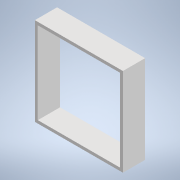
# Autodesk Inventor part: Верх
Saved by Autodesk Inventor 2021.2 (Build 252289000, 289)
## iProperties
Created: 2021-11-01
Part Number: Верх
Material: Типовые
Document SubType Name: Modeling
Designer: Kolan
Density: 1 g/cm^3
Appearance: По умолчанию
Author: Kolan
Autodesk Inventor part; units mm, degrees
ref_plane "YZ Plane" through (0, 0, 0) normal (1, 0, 0) x (0, 1, 0)
ref_plane "XZ Plane" through (0, 0, 0) normal (0, 1, 0) x (-1, 0, 0)
ref_plane "XY Plane" through (0, 0, 0) normal (0, 0, 1) x (1, 0, 0)
sketch "Эскиз1" plane through (0, 0, 0) normal (0, 0, 1) x (1, 0, 0)
  line L0 (41.178, 40.928) -> (-41.178, 40.928) construction
  line L1 (-41.178, 40.928) -> (-41.178, -40.928) construction
  line L2 (-41.178, -40.928) -> (41.178, -40.928) construction
  line L3 (41.178, -40.928) -> (41.178, 40.928) construction
  circle A0 centre (22.7283, 19.0964) radius 1 construction
  circle A1 centre (-19.4499, -22.8747) radius 1 construction
  circle A2 centre (19.3464, -22.9783) radius 1 construction
  line L4 (17.2251, 27.428) -> (22.7282, 21.9249) construction
  line L5 (22.7282, 21.9249) -> (19.8998, 19.0964) construction
  line L6 (19.8998, 19.0964) -> (22.7282, 16.268) construction
  line L7 (22.7282, 16.268) -> (25.5567, 19.0964) construction
  line L8 (25.5567, 19.0964) -> (27.678, 16.9751) construction
  line L9 (27.678, 16.9751) -> (27.678, -17.4751) construction
  line L10 (27.678, -17.4751) -> (22.1749, -22.9783) construction
  line L11 (22.1749, -22.9783) -> (19.3464, -20.1498) construction
  line L12 (19.3464, -20.1498) -> (16.518, -22.9783) construction
  line L13 (16.518, -22.9783) -> (19.3464, -25.8067) construction
  line L14 (19.3464, -25.8067) -> (17.2251, -27.928) construction
  line L15 (17.2251, -27.928) -> (-17.2251, -27.928) construction
  line L16 (-17.2251, -27.928) -> (-19.3464, -25.8067) construction
  line L17 (-19.3464, -25.8067) -> (-16.518, -22.9783) construction
  line L18 (-16.518, -22.9783) -> (-19.3464, -20.1498) construction
  line L19 (-19.3464, -20.1498) -> (-22.1749, -22.9783) construction
  line L20 (-22.1749, -22.9783) -> (-27.678, -17.4751) construction
  line L21 (-27.678, -17.4751) -> (-27.678, 16.9751) construction
  line L22 (-27.678, 16.9751) -> (-17.2251, 27.428) construction
  line L23 (-17.2251, 27.428) -> (17.2251, 27.428) construction
  line L24 (27.678, 27.428) -> (-27.678, 27.428)
  line L25 (-27.678, 27.428) -> (-27.678, -27.928)
  line L26 (-27.678, -27.928) -> (27.678, -27.928)
  line L27 (27.678, -27.928) -> (27.678, 27.428)
  line L28 (29.678, -29.928) -> (-29.678, -29.928)
  line L29 (-29.678, -29.928) -> (-29.678, 29.428)
  line L30 (-29.678, 29.428) -> (29.678, 29.428)
  line L31 (29.678, 29.428) -> (29.678, -29.928)
  point P0 (0, 0)
  dimension "d0" = 2
  constraints: 16 end point, 4 parallel, 2 perpendicular, 1 horizontal, 1 point on line, 3 other
  measures "d0" distance between parallel lines of L26 L28
extrude "Выдавливание1" add sketch "Эскиз1" along normal blind 10
sketch "Эскиз2" plane through (0, 0, 10) normal (0, 0, 1) x (1, 0, 0)
  line L0 (29.678, 29.428) -> (-29.678, 29.428) projected
  line L1 (-29.678, 29.428) -> (-29.678, -29.928) projected
  line L2 (29.678, 29.428) -> (-29.678, 29.428)
  line L3 (-29.678, 29.428) -> (-29.678, -29.928)
  line L4 (-29.678, -29.928) -> (29.678, -29.928)
  line L5 (29.678, -29.928) -> (29.678, 29.428)
  point P0 (0, 0)
  constraints: 8 end point, 2 parallel, 1 horizontal, 1 perpendicular
extrude "Выдавливание2" add sketch "Эскиз2" along normal blind 1.5
sketch "Эскиз3" plane through (0, 0, 10) normal (0, 0, -1) x (-1, 0, 0)
  line L0 (-27.678, 27.428) -> (-27.678, -27.928) construction
  line L1 (-27.678, -27.928) -> (27.678, -27.928) construction
  line L2 (27.678, -27.928) -> (27.678, 27.428) construction
  line L3 (27.678, 27.428) -> (-27.678, 27.428) construction
  line L4 (-29.678, -29.928) -> (-29.678, 29.428) construction
  line L5 (-29.678, -3.25) -> (-25.678, -3.25)
  line L6 (-25.678, -3.25) -> (-25.678, 2.75)
  line L7 (-25.678, 2.75) -> (-29.678, 2.75)
  line L8 (-29.678, 2.75) -> (-29.678, -3.25)
  line L9 (-27.678, 27.428) -> (-27.678, -27.928) construction
  line L10 (-27.678, -0.25) -> (27.678, -0.25) construction
  line L11 (0, -27.928) -> (0, 27.428) construction
  line L12 (29.678, -3.25) -> (25.678, -3.25)
  line L13 (25.678, -3.25) -> (25.678, 2.75)
  line L14 (25.678, 2.75) -> (29.678, 2.75)
  line L15 (29.678, 2.75) -> (29.678, -3.25)
  line L16 (-29.678, 29.428) -> (29.678, 29.428) construction
  line L17 (-3, 29.428) -> (3, 29.428)
  line L18 (3, 29.428) -> (3, 25.428)
  line L19 (3, 25.428) -> (-3, 25.428)
  line L20 (-3, 25.428) -> (-3, 29.428)
  line L21 (-3, -29.928) -> (3, -29.928)
  line L22 (3, -29.928) -> (3, -25.928)
  line L23 (3, -25.928) -> (-3, -25.928)
  line L24 (-3, -25.928) -> (-3, -29.928)
  point P0 (0, 0)
  dimension "d5" = 4
  dimension "d6" = 6
  dimension "d7" = 3
  dimension "d8" = 6
  dimension "d9" = 4
  dimension "d10" = 3
  constraints: 36 end point, 8 symmetric about line, 4 midpoint, 4 parallel, 2 horizontal, 2 perpendicular, 2 point on line
  measures "d5" distance of L7.end L6.end
  measures "d6" distance of L6.end L5.end
  measures "d7" distance from line of L10.start L7
  measures "d8" distance of L18.end L19.end
  measures "d9" distance of L17.end L18.end
  measures "d10" distance between parallel lines of L11 L18
extrude "Выдавливание3" add sketch "Эскиз3" along normal blind 20
sketch "Эскиз4" plane through (0, 0, 11.5) normal (0, 0, 1) x (1, 0, 0)
  line L0 (-10, -16.25) -> (5, -16.25)
  line L1 (5, -16.25) -> (5, 15.75)
  line L2 (5, 15.75) -> (-10, 15.75)
  line L3 (-10, 15.75) -> (-10, -16.25)
  line L4 (-29.678, 29.428) -> (-29.678, -29.928) construction
  point P0 (0, 0)
  point P1 (-29.678, -0.25)
  dimension "d13" = 15
  dimension "d14" = 32
  dimension "d15" = 16
  dimension "d16" = 5
  constraints: 8 end point, 2 parallel, 1 horizontal, 1 midpoint, 1 perpendicular
  measures "d13" distance of L2.end L1.end
  measures "d14" distance of L1.end L0.end
  measures "d15" distance from line of point (-29.678, -0.25) L2
  measures "d16" distance from line of point (0, 0) L1
extrude "Выдавливание4" cut sketch "Эскиз4" against normal through all
